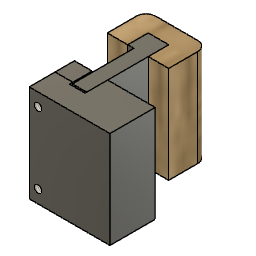
Lead Forming Die Set v11 (Autodesk Fusion 360 design; units mm, degrees)
Autodesk Fusion 360 part; units mm, degrees
note: some values were not read from the file. Set by a fixed rule: which sketch regions a step uses.
sketch "Sketch1" plane through (0, 0, 0) normal (0, 1, 0) x (1, 0, 0)
  line L0 (10.3, 0) -> (25, 0)
  line L1 (25, 0) -> (25, -14)
  line L2 (25, -14) -> (0, -14)
  line L3 (0, -14) -> (0, -6)
  line L4 (0, -6) -> (5.5, -6)
  line L5 (5.5, -6) -> (5.5, -7)
  line L6 (5.5, -7) -> (10.3, -7)
  line L7 (10.3, -7) -> (10.3, 0)
  dimension "d1" = 25
  dimension "d2" = 14
  dimension "d4" = 5.5
  dimension "d5" = 4.8
  dimension "d6" = 1
  dimension "d19" = 7
  dimension "d20" = 14
  constraint horizontal L0
  constraint vertical L1
  constraint horizontal L2
  constraint vertical L3
  constraint perpendicular L3 L4
  constraint perpendicular L4 L5
  constraint perpendicular L5 L6
  constraint perpendicular L0 L7
  measures "d1" distance of origin L0.end
  measures "d2" distance of origin L2.end
  measures "d4" distance of L3.end L4.end
  measures "d5" distance of L5.end L6.end
  measures "d6" distance of L4.end L5.end
  measures "d19" distance of L6.end L0.start
  measures "d20" distance of L0.end L1.end
extrude "Extrude1" add sketch "Sketch1" along normal blind 30 makes body 1
sketch "Sketch2" plane through (0, 0, 6) normal (0, 0, -1) x (-1, 0, 0)
  line L0 (-5.5, 0) -> (0, 0)
  line L1 (0, 0) -> (0, 30)
  line L2 (0, 30) -> (-5.5, 30)
  line L3 (-5.5, 30) -> (-5.5, 0)
  line L4 (-2.75, 0) -> (-2.75, 30) construction
  point P0 (-2.75, 4)
  point P1 (-2.75, 26)
  dimension "d9" = 4
  dimension "d10" = 4
  constraint midpoint L0 L4.start
  constraint midpoint L2 L4.end
  constraint coincident L4 P0
  constraint coincident L4 P1
  measures "d9" distance of L0 P0
  measures "d10" distance of L2 P1
hole "Hole1" at (2.75, 4, 6) at (2.75, 26, 6) direction (0, 0, 1) diameter 2.271 end through all bodies 1
thread "Thread1" "ANSI Unified Screw Threads 0.112(#4) 4-40 UNC 2B"
sketch "Sketch3" plane through (0, 0, 6) normal (0, 0, -1) x (-1, 0, 0)
  circle A0 centre (-2.75, 4) radius 1.1354
  circle A1 centre (-2.75, 26) radius 1.1354
  line L0 (-5.5, 0) -> (0, 0)
  line L1 (0, 0) -> (0, 30)
  line L2 (0, 30) -> (-5.5, 30)
  line L3 (-5.5, 30) -> (-5.5, 0)
  line L4 (-5.5, 0) -> (0, 0)
  line L5 (0, 0) -> (0, 30)
  line L6 (0, 30) -> (-5.5, 30)
  line L7 (-5.5, 30) -> (-5.5, 0)
  constraint horizontal L4
  constraint vertical L5
  constraint horizontal L6
  constraint vertical L7
  constraint coincident L1.end L2.start
  constraint coincident L0.start L3.end
extrude "Extrude2" add sketch "Sketch3" along normal blind 6 separate body makes body 2
sketch "Sketch4" plane through (0, 0, 0) normal (0, 0, -1) x (-1, 0, 0)
  circle A0 centre (-2.75, 4) radius 1.1354
  circle A1 centre (-2.75, 26) radius 1.1354
  line L0 (-5.5, 30) -> (-5.5, 0)
  line L1 (-5.5, 0) -> (0, 0)
  line L2 (0, 0) -> (0, 30)
  line L3 (0, 30) -> (-5.5, 30)
  point P0 (-2.75, 4)
  point P1 (-2.75, 26)
  constraint coincident P0 A0.centre
  constraint coincident P1 A1.centre
hole "Hole2" at (2.75, 4, 0) at (2.75, 26, 0) direction (0, 0, 1) diameter 3.264 depth 6 tip angle 180 bodies 2
sketch "Sketch5" plane through (0, 30, 0) normal (0, 1, 0) x (-1, 0, 0)
  line L0 (-10.3, 7) -> (-5.5, 7)
  line L1 (-5.5, 7) -> (-5.5, 6)
  line L2 (-5.5, 6) -> (0, 6)
  line L3 (0, 6) -> (0, 14)
  line L4 (0, 14) -> (-25, 14)
  line L5 (-25, 14) -> (-25, 0)
  line L6 (-25, 0) -> (-10.3, 0)
  line L7 (-10.3, 0) -> (-10.3, 7)
  line L8 (-10.3, 6.5) -> (-5.86, 6.5)
  line L9 (-5.86, 6.5) -> (-5.86, -12.55)
  line L10 (-10.3, -12.55) -> (-10.3, 6.5)
  line L11 (-5.86, -12.55) -> (-3.95, -12.55)
  line L12 (-3.95, -12.55) -> (-3.95, -18.9)
  line L13 (-3.95, -18.9) -> (-10.3, -18.9)
  line L14 (-10.3, -18.9) -> (-10.3, -12.55)
  dimension "d21" = 4.44
  dimension "d23" = 0.5
  dimension "d25" = 0.7
  dimension "d28" = 6.35
  dimension "d30" = 6.35
  dimension "d31" = 25.4
  constraint horizontal L8
  constraint vertical L9
  constraint vertical L10
  constraint coincident L7 L8.start
  constraint horizontal L11
  constraint vertical L12
  constraint horizontal L13
  constraint vertical L14
  measures "d21" distance of L8.start L8.end
  measures "d23" distance of L0 L8
  measures "d28" distance of L10.start L11.end
  measures "d30" distance of L11 L13
  measures "d31" distance of L8 L13
extrude "Extrude3" add sketch "Sketch5" against normal blind 30 separate body contours L7 L8 L9 L10 L11 L12 L13 L14 makes body 3
copy_body "Body->Comp1" bodies 1 removing the originals makes body 4 in component "Component"
copy_body "Body->Comp2" bodies 2 removing the originals makes body 5 in component "Component'"
copy_body "Body->Comp3" bodies 3 removing the originals makes body 6 in component "Component''"
sketch "Sketch6" plane through (0, 30, 0) normal (0, 1, 0) x (-1, 0, 0)
  line L0 (-10.3, 6.5) -> (-10.3, -18.9)
  line L1 (-10.3, -18.9) -> (-3.95, -18.9)
  line L2 (-3.95, -18.9) -> (-3.95, -12.55)
  line L3 (-3.95, -12.55) -> (-5.86, -12.55)
  line L4 (-5.86, -12.55) -> (-5.86, 6.5)
  line L5 (-5.86, 6.5) -> (-10.3, 6.5)
  line L6 (-3.95, -12.55) -> (-3.95, -18.9)
  line L7 (-10.3, -18.9) -> (-10.3, -12.55)
  line L8 (-10.3, -12.55) -> (-16.625, -12.55)
  line L9 (-16.625, -12.55) -> (-16.625, -21.55)
  line L10 (-13.625, -24.55) -> (-0.625, -24.55)
  line L11 (2.375, -21.55) -> (2.375, -12.55)
  line L12 (2.375, -12.55) -> (-3.95, -12.55)
  arc A0 (-0.625, -24.55) -> (2.375, -21.55) centre (-0.625, -21.55) ccw
  arc A1 (-16.625, -21.55) -> (-13.625, -24.55) centre (-13.625, -21.55) ccw
  point P0 (-16.625, -24.55)
  point P1 (2.375, -24.55)
  dimension "d32" = 6.35
  dimension "d33" = 19
  dimension "d34" = 6.325
  dimension "d35" = 12
  dimension "d36" = 3
  constraint coincident L2.end L3.start
  constraint coincident L1.end L2.start
  constraint coincident L0.end L1.start
  constraint perpendicular L1 L7
  constraint perpendicular L7 L8
  constraint perpendicular L1 L9
  constraint perpendicular L9 L10
  constraint perpendicular L10 L11
  constraint perpendicular L6 L12
  constraint coincident P1 L10
  constraint coincident P1 L11
  constraint tangent L10 A0
  constraint tangent L11 A0
  constraint coincident P0 L10
  constraint coincident P0 L9
  constraint tangent L10 A1
  constraint tangent L9 A1
  constraint equal A0 A1
  measures "d32" distance of L0.end L7.end
  measures "d33" distance of P0 P1
  measures "d34" distance of L6 L11
  measures "d35" distance of P1 L11.end
  measures "d36" radius of A0
extrude "Extrude4" add sketch "Sketch6" against normal up to surface (30 mm away) separate body contours L0 L1 L2 L6 L7 L8 L9 L10 L11 L12 A0 A1 makes body 7
copy_body "Body->Comp4" bodies 7 removing the originals makes body 8 in component "Component'''"
fillet "Fillet1" radius 0.6 2 edges at (10.3, 15, 6.5) (5.86, 15, 6.5) on bodies 6 in component "Component''"
component "Component" placed x (1, 0, 0) y (0, 1, 0) z (0, 0, 1) at (0, 0, 0)
component "Component'" placed x (1, 0, 0) y (0, 1, 0) z (0, 0, 1) at (0, 0, 0)
component "Component''" placed x (1, 0, 0) y (0, 1, 0) z (0, 0, 1) at (0, 0, 0)
component "Component'''" placed x (1, 0, 0) y (0, 1, 0) z (0, 0, 1) at (0, 0, 0)
equation "d34 = ( ( 19 - 6.35 ) / 2 ) * 1 mm"
